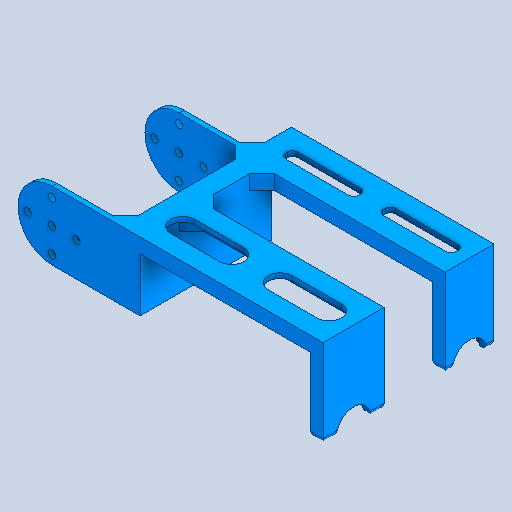
# Autodesk Inventor part: Claw1
Saved by Autodesk Inventor 2023 (Build 270158000, 158)
## iProperties
Created: 2020-01-09
Part Number: Claw1
Material: 일반
Document SubType Name: Modeling
Designer: Knowblesse
Density: 1 g/cm^3
Appearance: 기본값
Author: Knowblesse
Autodesk Inventor part; units mm, degrees
ref_plane "YZ Plane" through (0, 0, 0) normal (1, 0, 0) x (0, 1, 0)
ref_plane "XZ Plane" through (0, 0, 0) normal (0, 1, 0) x (-1, 0, 0)
ref_plane "XY Plane" through (0, 0, 0) normal (0, 0, 1) x (1, 0, 0)
sketch "스케치1" plane through (0, 0, 0) normal (0, 0, 1) x (1, 0, 0)
  line L0 (0, 0) -> (50, 0)
  line L1 (50, 0) -> (50, 28)
  line L2 (50, 28) -> (0, 28)
  line L3 (0, 28) -> (0, 0)
  circle A0 centre (14, 14) radius 14
  line L4 (0, 14) -> (50, 14) construction
  point P0 (14, 0)
  point P1 (14, 28)
  dimension "d0" = 36
  dimension "d1" = 28
  constraints: 10 end point, 2 midpoint, 2 parallel, 2 tangent, 1 centre point, 1 horizontal, 1 perpendicular, 1 point on line
  measures "d0" distance from line of L1 A0.centre
  measures "d1" diameter of A0
extrude "돌출1" add sketch "스케치1" along normal blind 54 contours A0 L2 L1 L0 | A0
sketch "스케치2" plane through (14, 28, 0) normal (0, 1, 0) x (1, 0, 0)
  line L0 (0, 0) -> (0, 0) projected
  line L1 (0, 0) -> (0, -54) projected
  line L2 (0, -54) -> (0, -54) projected
  line L3 (0, 0) -> (0, -54) projected
  line L4 (36, 0) -> (0, 0) projected
  line L5 (0, 0) -> (0, -54) projected
  line L6 (36, -54) -> (0, -54) projected
  line L7 (36, 0) -> (36, -54) projected
  line L8 (-14, -2) -> (28, -2)
  line L9 (28, -2) -> (28, -52)
  line L10 (28, -52) -> (-14, -52)
  line L11 (-14, -52) -> (-14, -2)
  line L12 (-14, 0) -> (0, 0) projected
  line L13 (36, 0) -> (36, -54) projected
  dimension "d4" = 2
  dimension "d5" = 2
  dimension "d6" = 8
  constraints: 8 end point, 2 parallel, 1 horizontal, 1 perpendicular, 1 vertical alignment
  measures "d4" distance between parallel lines of L4 L8
  measures "d5" distance between parallel lines of L6 L10
  measures "d6" distance between parallel lines of L13 L9
extrude "돌출2" cut sketch "스케치2" against normal up to surface (28 mm away) contours L8 L9 L10 L1 | L1 L10 L11 L8
sketch "스케치3" plane through (0, 0, 0) normal (0, 0, -1) x (-1, 0, 0)
  line L0 (-50, 0) -> (-50, 28) projected
  line L1 (-14, 0) -> (-50, 0) projected
  arc A0 (-14, 0) -> (-14, 28) centre (-14, 14) ccw projected
  line L2 (-50, 28) -> (-14, 28) projected
  point P0 (0, 0)
  point P1 (-14, 24)
  point P2 (-24, 14)
  point P3 (-14, 4)
  point P4 (-4, 14)
  dimension "d9" = 10
  dimension "d12" = 360
  constraints: 1 vertical alignment, 5 other
  measures "d9" distance of point (-14, 24) A0.centre
hole "구멍1" at (14, 24, 0) at (24, 14, 0) at (14, 4, 0) at (4, 14, 0) at (14, 14, 0) direction (0, 0, 1) diameter 3 end through all
sketch "스케치4" plane through (14, 28, 0) normal (0, 1, 0) x (1, 0, 0)
  line L0 (28, -52) -> (0, -52) projected
  line L1 (0, -52) -> (0, -54) projected
  line L2 (36, -54) -> (0, -54) projected
  line L3 (36, 0) -> (36, -54) projected
  line L4 (36, 0) -> (0, 0) projected
  line L5 (0, 0) -> (0, -2) projected
  line L6 (0, -2) -> (28, -2) projected
  line L7 (28, -2) -> (28, -52) projected
  line L8 (28, -54) -> (111, -54)
  line L9 (111, -54) -> (111, -29)
  line L10 (111, -29) -> (28, -29)
  line L11 (28, -29) -> (28, -54)
  line L12 (28, -4) -> (111, -4)
  line L13 (111, -4) -> (111, 16)
  line L14 (111, 16) -> (28, 16)
  line L15 (28, 16) -> (28, -4)
  line L16 (46, -29) -> (46, -4)
  line L17 (28, -41.5) -> (111, -41.5) construction
  line L18 (111, 6) -> (28, 6) construction
  line L19 (41, -46.5) -> (61, -46.5)
  line L20 (66, -41.5) -> (66, -41.5)
  line L21 (61, -36.5) -> (41, -36.5)
  line L22 (36, -41.5) -> (36, -41.5)
  line L23 (81, -46.5) -> (101, -46.5)
  line L24 (106, -41.5) -> (106, -41.5)
  line L25 (101, -36.5) -> (81, -36.5)
  line L26 (76, -41.5) -> (76, -41.5)
  line L27 (38, 3.5) -> (64, 3.5)
  line L28 (66, 5.5) -> (66, 6.5)
  line L29 (64, 8.5) -> (38, 8.5)
  line L30 (36, 6.5) -> (36, 5.5)
  line L31 (78, 3.5) -> (104, 3.5)
  line L32 (106, 5.5) -> (106, 6.5)
  line L33 (104, 8.5) -> (78, 8.5)
  line L34 (76, 6.5) -> (76, 5.5)
  arc A0 (38, 8.5) -> (36, 6.5) centre (38, 6.5) ccw
  arc A1 (36, 5.5) -> (38, 3.5) centre (38, 5.5) ccw
  arc A2 (66, 6.5) -> (64, 8.5) centre (64, 6.5) ccw
  arc A3 (64, 3.5) -> (66, 5.5) centre (64, 5.5) ccw
  arc A4 (76, 5.5) -> (78, 3.5) centre (78, 5.5) ccw
  arc A5 (78, 8.5) -> (76, 6.5) centre (78, 6.5) ccw
  arc A6 (106, 6.5) -> (104, 8.5) centre (104, 6.5) ccw
  arc A7 (104, 3.5) -> (106, 5.5) centre (104, 5.5) ccw
  arc A8 (41, -36.5) -> (36, -41.5) centre (41, -41.5) ccw
  arc A9 (66, -41.5) -> (61, -36.5) centre (61, -41.5) ccw
  arc A10 (61, -46.5) -> (66, -41.5) centre (61, -41.5) ccw
  arc A11 (36, -41.5) -> (41, -46.5) centre (41, -41.5) ccw
  arc A12 (76, -41.5) -> (81, -46.5) centre (81, -41.5) ccw
  arc A13 (81, -36.5) -> (76, -41.5) centre (81, -41.5) ccw
  arc A14 (106, -41.5) -> (101, -36.5) centre (101, -41.5) ccw
  arc A15 (101, -46.5) -> (106, -41.5) centre (101, -41.5) ccw
  point P0 (66, -36.5)
  point P1 (66, -46.5)
  point P2 (36, -36.5)
  point P3 (76, -46.5)
  point P4 (106, -36.5)
  point P5 (106, -46.5)
  point P6 (76, -36.5)
  point P7 (66, 8.5)
  point P8 (66, 3.5)
  point P9 (36, 8.5)
  point P10 (76, 3.5)
  point P11 (106, 8.5)
  point P12 (106, 3.5)
  point P13 (76, 8.5)
  point P14 (66, -41.5)
  point P15 (36, 6)
  point P16 (36, -41.5)
  point P17 (36, -41.5)
  point P18 (36, -41.5)
  point P19 (36, -29)
  point P20 (28, 0)
  point P21 (36, -4)
  dimension "d78" = 83
  dimension "d79" = 25
  dimension "d80" = 20
  dimension "d81" = 25
  dimension "d82" = 10
  dimension "d83" = 30
  dimension "d84" = 10
  dimension "d85" = 30
  dimension "d86" = 10
  dimension "d87" = 30
  dimension "d88" = 5
  dimension "d89" = 30
  dimension "d90" = 5
  dimension "d91" = 5
  dimension "d92" = 2
  dimension "d93" = 5
  constraints: 54 end point, 37 point on line, 32 point on circle, 32 tangent, 16 centre point, 14 equal radius, 12 parallel, 7 perpendicular, 6 horizontal, 6 midpoint, 4 collinear
  measures "d78" distance of L10.end L9.end
  measures "d79" distance of L9.end L8.end
  measures "d80" distance of L13.end L12.end
  measures "d81" distance between parallel lines of L12 L10
  measures "d82" distance between parallel lines of L3 L16
  measures "d83" distance of point (36, -36.5) point (66, -36.5)
  measures "d84" distance of point (66, -36.5) point (66, -46.5)
  measures "d85" distance of point (76, -36.5) point (106, -36.5)
  measures "d86" distance of point (106, -36.5) point (106, -46.5)
  measures "d87" distance of point (36, 8.5) point (66, 8.5)
  measures "d88" distance of point (66, 8.5) point (66, 3.5)
  measures "d89" distance of point (76, 8.5) point (106, 8.5)
  measures "d90" distance of point (106, 8.5) point (106, 3.5)
  measures "d91" distance between parallel lines of L13 L32
  measures "d92" radius of A0
  measures "d93" radius of A8
extrude "돌출3" add sketch "스케치4" against normal blind 2 contours L10 L9 L8 L3 | L3 L4 L15 L14 L13 L12
sketch "스케치5" plane through (14, 26, 0) normal (0, -1, 0) x (1, 0, 0)
  line L0 (28, 0) -> (36, 0) projected
  line L1 (36, 41.5) -> (36, 54) projected
  line L2 (61, 36.5) -> (41, 36.5) projected
  arc A0 (36, 41.5) -> (41, 36.5) centre (41, 41.5) ccw projected
  line L3 (36, 29) -> (36, 41.5) projected
  line L4 (36, 29) -> (111, 29) projected
  line L5 (111, 29) -> (111, 54) projected
  line L6 (111, 54) -> (36, 54) projected
  arc A1 (41, 46.5) -> (36, 41.5) centre (41, 41.5) ccw projected
  line L7 (41, 46.5) -> (61, 46.5) projected
  arc A2 (61, 36.5) -> (61, 46.5) centre (61, 41.5) ccw projected
  line L8 (28, 0) -> (28, -16) projected
  line L9 (28, -16) -> (111, -16) projected
  line L10 (111, -16) -> (111, 4) projected
  line L11 (111, 4) -> (36, 4) projected
  line L12 (36, 0) -> (36, 4) projected
  line L13 (111, 29) -> (111, 54) projected
  line L14 (36, 41.5) -> (36, 54) projected
  line L15 (111, 54) -> (36, 54)
  line L16 (36, 54) -> (36, 51.5)
  line L17 (36, 51.5) -> (111, 51.5)
  line L18 (111, 51.5) -> (111, 54)
  line L19 (111, 29) -> (36, 29) projected
  line L20 (36, 29) -> (36, 41.5) projected
  line L21 (111, 29) -> (36, 29)
  line L22 (36, 29) -> (36, 33)
  line L23 (36, 33) -> (111, 33)
  line L24 (111, 33) -> (111, 29)
  line L25 (111, 4) -> (36, 4) projected
  line L26 (28, 0) -> (28, -16) projected
  line L27 (111, 4) -> (28, 4)
  line L28 (28, 4) -> (28, 0)
  line L29 (28, 0) -> (111, 0)
  line L30 (111, 0) -> (111, 4)
  line L31 (30.5, 0) -> (30.5, -13.5)
  line L32 (30.5, -13.5) -> (111, -13.5)
  line L33 (111, -16) -> (111, 4) projected
  point P0 (-14, 0)
  point P1 (36, 33)
  point P2 (36, 51.5)
  point P3 (30.5, 0)
  dimension "d94" = 2.5
  dimension "d95" = 4
  dimension "d96" = 4
  dimension "d97" = 2.5
  dimension "d98" = 2.5
  constraints: 28 end point, 6 parallel, 5 perpendicular, 5 point on line, 3 horizontal
  measures "d94" distance of L16.end L15.end
  measures "d95" distance of L21.end L22.end
  measures "d96" distance of L28.end L27.end
  measures "d97" distance between parallel lines of L8 L31
  measures "d98" distance between parallel lines of L32 L9
extrude "돌출4" add sketch "스케치5" along normal blind 4 contours L28 L27 L12 L0 | L0 L31 L32 L10 L9 L8 | L12 L11 L10 L29 | L1 L6 L5 L17 | L23 L5 L4 L3
sketch "스케치6" plane through (14, 26, 0) normal (0, -1, 0) x (1, 0, 0)
  line L0 (0, 54) -> (111, 54) projected
  line L1 (28, 0) -> (0, 0) projected
  line L2 (0, 0) -> (0, 2) projected
  line L3 (0, 2) -> (28, 2) projected
  line L4 (28, 52) -> (0, 52) projected
  line L5 (0, 52) -> (0, 54) projected
  line L6 (28, 2) -> (28, 52) projected
  line L7 (111, 54) -> (111, 29) projected
  line L8 (111, 29) -> (36, 29) projected
  line L9 (36, 4) -> (36, 29) projected
  line L10 (36, 4) -> (111, 4) projected
  line L11 (111, 4) -> (111, -16) projected
  line L12 (111, -16) -> (28, -16) projected
  line L13 (28, -16) -> (28, 0) projected
  line L14 (111, 54) -> (111, 29) projected
  line L15 (111, 29) -> (36, 29) projected
  line L16 (111, 54) -> (106, 54)
  line L17 (106, 54) -> (106, 29)
  line L18 (106, 29) -> (111, 29)
  line L19 (111, 29) -> (111, 54)
  line L20 (111, 4) -> (111, -16) projected
  line L21 (111, -16) -> (28, -16) projected
  line L22 (111, 4) -> (106, 4)
  line L23 (106, 4) -> (106, -16)
  line L24 (106, -16) -> (111, -16)
  line L25 (111, -16) -> (111, 4)
  dimension "d99" = 5
  constraints: 16 end point, 4 parallel, 3 point on line, 2 horizontal, 2 perpendicular
  measures "d99" distance of L18.end L17.end
extrude "돌출5" add sketch "스케치6" along normal blind 34 contours L0 L7 L8 L17 | L10 L11 L12 L23
sketch "스케치10" plane through (125, 28, 54) normal (1, 0, 0) x (0, 0, -1)
  line L0 (25, 0) -> (25, -36) projected
  line L1 (0, 0) -> (25, 0) projected
  line L2 (0, 0) -> (0, -36) projected
  line L3 (25, -36) -> (0, -36) projected
  line L4 (50, 0) -> (50, -36) projected
  line L5 (70, -36) -> (50, -36) projected
  line L6 (70, 0) -> (70, -36) projected
  line L7 (50, 0) -> (70, 0) projected
  circle A0 centre (12.5, -36) radius 7
  line L8 (70, -36) -> (50, -36) projected
  circle A1 centre (60, -36) radius 7
  point P0 (54, -28)
  point P1 (53, -36)
  point P2 (67, -36)
  point P3 (5.5, -36)
  point P4 (19.5, -36)
  dimension "d100" = 14
  dimension "d101" = 14
  constraints: 2 centre point, 2 midpoint
  measures "d100" diameter of A0
  measures "d101" diameter of A1
extrude "돌출8" cut sketch "스케치10" against normal up to surface (5 mm away) contours L3 A0 | A1 L5 picked at (14.446, -32.81) picked at (60.8274, -33.8183)
chamfer "모따기1" distance 5 angle 45 7 edges at (42, 14, 52) (42, 14, 2) (42, 25, 0) (50, 25, 29) (50, 25, 4) (50, 24, 51.5) (50, 24, 33)
chamfer "모따기2" distance 5 angle 45 3 edges at (39.5, 22, 0) (43.25, 22, 0) (44.5, 24, 0)
sketch "스케치11" plane through (14, -8, 0) normal (0, -1, 0) x (1, 0, 0)
  line L0 (36, 38) -> (41, 33) projected
  line L1 (41, 33) -> (106, 33) projected
  line L2 (106, 33) -> (106, 41.5) projected
  arc A0 (101, 36.5) -> (106, 41.5) centre (101, 41.5) ccw projected
  line L3 (101, 36.5) -> (81, 36.5) projected
  arc A1 (81, 46.5) -> (81, 36.5) centre (81, 41.5) ccw projected
  line L4 (81, 46.5) -> (101, 46.5) projected
  arc A2 (106, 41.5) -> (101, 46.5) centre (101, 41.5) ccw projected
  line L5 (106, 41.5) -> (106, 51.5) projected
  line L6 (106, 51.5) -> (41, 51.5) projected
  line L7 (41, 51.5) -> (36, 46.5) projected
  line L8 (36, 41.5) -> (36, 46.5) projected
  arc A3 (41, 46.5) -> (36, 41.5) centre (41, 41.5) ccw projected
  line L9 (41, 46.5) -> (61, 46.5) projected
  arc A4 (61, 36.5) -> (61, 46.5) centre (61, 41.5) ccw projected
  line L10 (61, 36.5) -> (41, 36.5) projected
  arc A5 (36, 41.5) -> (41, 36.5) centre (41, 41.5) ccw projected
  line L11 (36, 38) -> (36, 41.5) projected
  line L12 (106, 41.5) -> (106, 51.5) projected
  line L13 (106, 51.5) -> (108, 51.5)
  line L14 (108, 51.5) -> (108, 33)
  line L15 (108, 33) -> (106, 33)
  line L16 (106, 33) -> (106, 51.5)
  line L17 (35.5, 0) -> (30.5, -5) projected
  line L18 (30.5, -5) -> (30.5, -13.5) projected
  line L19 (30.5, -13.5) -> (106, -13.5) projected
  line L20 (106, -13.5) -> (106, -6.5) projected
  arc A6 (104, -8.5) -> (106, -6.5) centre (104, -6.5) ccw projected
  line L21 (104, -8.5) -> (78, -8.5) projected
  arc A7 (76, -6.5) -> (78, -8.5) centre (78, -6.5) ccw projected
  line L22 (76, -6.5) -> (76, -5.5) projected
  arc A8 (78, -3.5) -> (76, -5.5) centre (78, -5.5) ccw projected
  line L23 (78, -3.5) -> (104, -3.5) projected
  arc A9 (106, -5.5) -> (104, -3.5) centre (104, -5.5) ccw projected
  line L24 (106, -5.5) -> (106, 0) projected
  line L25 (106, 0) -> (35.5, 0) projected
  line L26 (36, -6.5) -> (36, -5.5) projected
  arc A10 (38, -3.5) -> (36, -5.5) centre (38, -5.5) ccw projected
  line L27 (38, -3.5) -> (64, -3.5) projected
  arc A11 (66, -5.5) -> (64, -3.5) centre (64, -5.5) ccw projected
  line L28 (66, -5.5) -> (66, -6.5) projected
  arc A12 (64, -8.5) -> (66, -6.5) centre (64, -6.5) ccw projected
  line L29 (64, -8.5) -> (38, -8.5) projected
  arc A13 (36, -6.5) -> (38, -8.5) centre (38, -6.5) ccw projected
  line L30 (106, -5.5) -> (106, 0) projected
  line L31 (106, 0) -> (108, 0)
  line L32 (108, 0) -> (108, -13.5)
  line L33 (108, -13.5) -> (106, -13.5)
  line L34 (106, -13.5) -> (106, 0)
  point P0 (-14, 0)
  point P1 (106, -5.5)
  dimension "d104" = 2
  dimension "d105" = 2
  constraints: 16 end point, 4 parallel, 2 collinear, 2 horizontal, 2 perpendicular
  measures "d104" distance of L14.end L15.end
  measures "d105" distance of L32.end L33.end
extrude "돌출9" cut sketch "스케치11" against normal up to surface (34 mm away) contours L2 L5 L13 L14 L15 | L31 L32 L33 L20 L34 L24
fillet "모깎기1" radius 2 14 edges at (125, -8, 51.25) (122.5, -8, 54) (120, -8, 52.75) (123.5, -8, 48.5) (123.5, -8, 34.5) (125, -8, 31.75) (122.5, -8, 29) (120, -8, 31) (120, -8, 2.5) (122.5, -8, 4) (125, -8, 2.5) (120, -8, -14.75) (122.5, -8, -16) (125, -8, -14.5)
chamfer "모따기3" distance 5 angle 45 2 edges at (122, 26, 42.25) (122, 26, -6.75)
